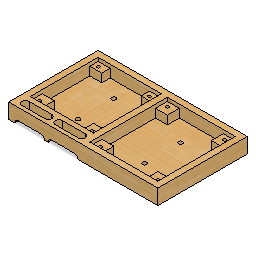
Electronics V8 case (Autodesk Fusion 360 design; units mm, degrees)
Autodesk Fusion 360 part; units mm, degrees
note: some values were not read from the file. Chosen so that the rebuilt part matches the saved one: which face or edge a step refers to.
box "BoxPrimitive1" add length 74.75 width 124.7 height 12.7 placed x (0, 0, -1) y (-1, 0, 0) z (0, 1, 0) at (0, 0, 0) makes body 1
copy_body "CutPasteBodies1" bodies 1 removing the originals makes body 2 in component "Stock"
box "BoxPrimitive1'" add length 52.9 width 56.75 height 8 placed x (0, 0, -1) y (-1, 0, 0) z (0, 1, 0) at (-15.6378, 0, 82.7892) separate body makes body 3 in component "Smaller cutout"
move_body "Move1" bodies 3 to x (1, 0, 0) y (0, 1, 0) z (0, 0, 1) at (-52.3122, 4.7, -82.7892) in component "Smaller cutout"
move_body "Move2" bodies 3 to x (1, 0, 0) y (0, 1, 0) z (0, 0, 1) at (-50, 0, 0) in component "Smaller cutout"
move_body "Move3" bodies 3 to x (1, 0, 0) y (0, 1, 0) z (0, 0, 1) at (50, 0, -21.85) in component "Smaller cutout"
move_body "Move4" bodies 3 to x (1, 0, 0) y (0, 1, 0) z (0, 0, 1) at (5, 0, 5) in component "Smaller cutout"
box "BoxPrimitive1''" add length 64.75 width 56.8 height 5 placed x (0, 0, -1) y (-1, 0, 0) z (0, 1, 0) at (-52.8442, 0, 39.9894) separate body makes body 4 in component "Bigger cutout"
move_body "Move1'" bodies 4 to x (1, 0, 0) y (0, 1, 0) z (0, 0, 1) at (46.6942, 7.7, -44.9894) in component "Bigger cutout"
move_body "Move2'" bodies 4 to x (1, 0, 0) y (0, 1, 0) z (0, 0, 1) at (5, 0, 0) in component "Bigger cutout"
move_body "Move5" bodies 3 to x (0, 0, -1) y (0, 1, 0) z (1, 0, 0) at (-49.95, 0, -189.45) in component "Smaller cutout"
move_body "Move6" bodies 3 to x (1, 0, 0) y (0, 1, 0) z (0, 0, 1) at (-5, 0, 51.75) in component "Smaller cutout"
move_body "Move7" bodies 3 to x (1, 0, 0) y (0, 1, 0) z (0, 0, 1) at (5, 0, 5) in component "Smaller cutout"
move_body "Move3'" bodies 4 to x (1, 0, 0) y (0, 1, 0) z (0, 0, 1) at (-8.85, 0, 0) in component "Bigger cutout"
move_body "Move4'" bodies 4 to x (1, 0, 0) y (0, 1, 0) z (0, 0, 1) at (5, 0, 0) in component "Bigger cutout"
move_face "OffsetFaces1" offset 5 1 faces at (-42.8667, 7.7, -26.5833) on bodies 4 in component "Bigger cutout"
cylinder "CylinderPrimitive1" add diameter 2.5 height 12.7 placed x (1, 0, 0) y (0, 0, -1) z (0, 1, 0) at (-30.8242, 0, 13.5156) separate body makes body 5 in component "PCB screw holes"
copy_body "CopyPasteBodies1" bodies 5 makes body 6 in component "PCB screw holes"
move_body "Move1''" bodies 6 to x (1, 0, 0) y (0, 1, 0) z (0, 0, 1) at (15, 0, 0) in component "PCB screw holes"
copy_body "CopyPasteBodies2" bodies 5 makes body 7 in component "PCB screw holes"
move_body "Move2''" bodies 7 to x (1, 0, 0) y (0, 1, 0) z (0, 0, 1) at (-25, 0, 0) in component "PCB screw holes"
copy_body "CopyPasteBodies3" bodies 5 makes body 8 in component "PCB screw holes"
move_body "Move3''" bodies 8 to x (1, 0, 0) y (0, 1, 0) z (0, 0, 1) at (-50, 0, 0) in component "PCB screw holes"
copy_body "CopyPasteBodies4" bodies 5 makes body 9 in component "PCB screw holes"
move_body "Move4''" bodies 9 to x (1, 0, 0) y (0, 1, 0) z (0, 0, 1) at (-65, 0, 0) in component "PCB screw holes"
copy_body "CopyPasteBodies5" bodies 5 makes body 10 in component "PCB screw holes"
move_body "Move5'" bodies 10 to x (1, 0, 0) y (0, 1, 0) z (0, 0, 1) at (-85, 0, 0) in component "PCB screw holes"
copy_body "CopyPasteBodies6" bodies 5 makes body 11 in component "PCB screw holes"
move_body "Move6'" bodies 11 to x (1, 0, 0) y (0, 1, 0) z (0, 0, 1) at (-105, 0, 0) in component "PCB screw holes"
copy_body "CopyPasteBodies7" bodies 5 makes body 12 in component "PCB screw holes"
move_body "Move7'" bodies 12 to x (1, 0, 0) y (0, 1, 0) z (0, 0, 1) at (30, 0, 0) in component "PCB screw holes"
move_body "Move8" bodies 5 to x (1, 0, 0) y (0, 1, 0) z (0, 0, 1) at (-88.8758, 0, -83.2656) in component "PCB screw holes"
move_body "Move9" bodies 5 to x (1, 0, 0) y (0, 1, 0) z (0, 0, 1) at (3.9, 0, 0) in component "PCB screw holes"
move_body "Move10" bodies 5 to x (1, 0, 0) y (0, 1, 0) z (0, 0, 1) at (0, 0, 3.9) in component "PCB screw holes"
move_body "Move11" bodies 6 to x (1, 0, 0) y (0, 1, 0) z (0, 0, 1) at (-103.8758, 0, -26.5156) in component "PCB screw holes"
move_body "Move12" bodies 6 to x (1, 0, 0) y (0, 1, 0) z (0, 0, 1) at (3.9, 0, 0) in component "PCB screw holes"
move_body "Move13" bodies 6 to x (1, 0, 0) y (0, 1, 0) z (0, 0, 1) at (0, 0, -3.9) in component "PCB screw holes"
move_body "Move14" bodies 7 to x (1, 0, 0) y (0, 1, 0) z (0, 0, 1) at (-10.9758, 0, -83.2656) in component "PCB screw holes"
move_body "Move15" bodies 7 to x (1, 0, 0) y (0, 1, 0) z (0, 0, 1) at (-5.1, 0, 3.9) in component "PCB screw holes"
move_body "Move16" bodies 8 to x (1, 0, 0) y (0, 1, 0) z (0, 0, 1) at (14.0242, 0, -26.5156) in component "PCB screw holes"
move_body "Move17" bodies 8 to x (1, 0, 0) y (0, 1, 0) z (0, 0, 1) at (-5.1, 0, -3.9) in component "PCB screw holes"
move_body "Move18" bodies 9 to x (1, 0, 0) y (0, 1, 0) z (0, 0, 1) at (34.0242, 0, -83.2656) in component "PCB screw holes"
move_body "Move19" bodies 9 to x (1, 0, 0) y (0, 1, 0) z (0, 0, 1) at (3.9, 0, 3.9) in component "PCB screw holes"
move_body "Move20" bodies 10 to x (1, 0, 0) y (0, 1, 0) z (0, 0, 1) at (54.0242, 0, -18.5156) in component "PCB screw holes"
move_body "Move21" bodies 10 to x (1, 0, 0) y (0, 1, 0) z (0, 0, 1) at (3.9, 0, -3.9) in component "PCB screw holes"
move_body "Move22" bodies 11 to x (1, 0, 0) y (0, 1, 0) z (0, 0, 1) at (130.8242, 0, -83.2656) in component "PCB screw holes"
move_body "Move23" bodies 11 to x (1, 0, 0) y (0, 1, 0) z (0, 0, 1) at (-3.9, 0, 3.9) in component "PCB screw holes"
move_body "Move24" bodies 12 to x (1, 0, 0) y (0, 1, 0) z (0, 0, 1) at (-4.1758, 0, -18.5156) in component "PCB screw holes"
move_body "Move25" bodies 12 to x (1, 0, 0) y (0, 1, 0) z (0, 0, 1) at (-3.9, 0, -3.9) in component "PCB screw holes"
move_face "OffsetFaces1'" offset 2 1 faces at (-102.0667, 4.7, -31.9167) on bodies 3 in component "Smaller cutout"
box "BoxPrimitive2" add length 10 width 10 height 7 placed x (0, 0, -1) y (-1, 0, 0) z (0, 1, 0) at (-122.8706, 0, 22.3895) separate body makes body 13 in component "PCB supports"
copy_body "CopyPasteBodies9" bodies 13 makes body 14 in component "PCB supports"
move_body "Move12'" bodies 14 to x (1, 0, 0) y (0, 1, 0) z (0, 0, 1) at (20, 0, 0) in component "PCB supports"
copy_body "CopyPasteBodies10" bodies 13 makes body 15 in component "PCB supports"
move_body "Move13'" bodies 15 to x (1, 0, 0) y (0, 1, 0) z (0, 0, 1) at (35, 0, 0) in component "PCB supports"
copy_body "CopyPasteBodies11" bodies 13 makes body 16 in component "PCB supports"
move_body "Move14'" bodies 16 to x (1, 0, 0) y (0, 1, 0) z (0, 0, 1) at (50, 0, 0) in component "PCB supports"
copy_body "CopyPasteBodies12" bodies 13 makes body 17 in component "PCB supports"
move_body "Move15'" bodies 17 to x (1, 0, 0) y (0, 1, 0) z (0, 0, 1) at (0, 0, -20) in component "PCB supports"
copy_body "CopyPasteBodies13" bodies 13 makes body 18 in component "PCB supports"
move_body "Move16'" bodies 18 to x (1, 0, 0) y (0, 1, 0) z (0, 0, 1) at (0, 0, -40) in component "PCB supports"
copy_body "CopyPasteBodies14" bodies 13 makes body 19 in component "PCB supports"
move_body "Move17'" bodies 19 to x (1, 0, 0) y (0, 1, 0) z (0, 0, 1) at (0, 0, -60) in component "PCB supports"
copy_body "CopyPasteBodies15" bodies 13 makes body 20 in component "PCB supports"
move_body "Move18'" bodies 20 to x (1, 0, 0) y (0, 1, 0) z (0, 0, 1) at (0, 0, -80) in component "PCB supports"
move_body "Move19'" bodies 20 to x (1, 0, 0) y (0, 1, 0) z (0, 0, 1) at (-20, 0, 0) in component "PCB supports"
move_body "Move20'" bodies 20 to x (1, 0, 0) y (0, 1, 0) z (0, 0, 1) at (33.1706, 2.7, -2.1395) in component "PCB supports"
move_body "Move21'" bodies 19 to x (1, 0, 0) y (0, 1, 0) z (0, 0, 1) at (13.1706, 2.7, 24.6105) in component "PCB supports"
move_body "Move22'" bodies 18 to x (1, 0, 0) y (0, 1, 0) z (0, 0, 1) at (56.0706, 2.7, 4.6105) in component "PCB supports"
move_body "Move23'" bodies 17 to x (1, 0, 0) y (0, 1, 0) z (0, 0, 1) at (56.0706, 2.7, -62.1395) in component "PCB supports"
move_body "Move24'" bodies 13 to x (1, 0, 0) y (0, 1, 0) z (0, 0, 1) at (71.0706, 2.7, -27.3895) in component "PCB supports"
move_body "Move25'" bodies 14 to x (1, 0, 0) y (0, 1, 0) z (0, 0, 1) at (51.0706, 2.7, -82.1395) in component "PCB supports"
move_body "Move26" bodies 16 to x (1, 0, 0) y (0, 1, 0) z (0, 0, 1) at (67.8706, 2.7, -27.3895) in component "PCB supports"
move_body "Move27" bodies 15 to x (1, 0, 0) y (0, 1, 0) z (0, 0, 1) at (82.8706, 2.7, -82.1395) in component "PCB supports"
cylinder "CylinderPrimitive1'" add diameter 3.5 height 12.7 placed x (1, 0, 0) y (0, 0, -1) z (0, 1, 0) at (-133.1666, 0, 19.1223) separate body makes body 21 in component "Mounting screw holes"
copy_body "CopyPasteBodies1'" bodies 21 makes body 22 in component "Mounting screw holes"
move_body "Move1'''" bodies 22 to x (1, 0, 0) y (0, 1, 0) z (0, 0, 1) at (25, 0, 0) in component "Mounting screw holes"
copy_body "CopyPasteBodies2'" bodies 21 makes body 23 in component "Mounting screw holes"
move_body "Move2'''" bodies 23 to x (1, 0, 0) y (0, 1, 0) z (0, 0, 1) at (45, 0, 0) in component "Mounting screw holes"
copy_body "CopyPasteBodies3'" bodies 21 makes body 24 in component "Mounting screw holes"
move_body "Move3'''" bodies 24 to x (1, 0, 0) y (0, 1, 0) z (0, 0, 1) at (75, 0, 0) in component "Mounting screw holes"
move_body "Move4'''" bodies 21 to x (1, 0, 0) y (0, 1, 0) z (0, 0, 1) at (39.9166, 0, -60.4973) in component "Mounting screw holes"
move_body "Move5''" bodies 21 to x (1, 0, 0) y (0, 1, 0) z (0, 0, 1) at (0, 0, -15) in component "Mounting screw holes"
move_body "Move6''" bodies 22 to x (1, 0, 0) y (0, 1, 0) z (0, 0, 1) at (14.9166, 0, -60.4973) in component "Mounting screw holes"
move_body "Move7''" bodies 22 to x (1, 0, 0) y (0, 1, 0) z (0, 0, 1) at (0, 0, 15) in component "Mounting screw holes"
move_body "Move8'" bodies 23 to x (1, 0, 0) y (0, 1, 0) z (0, 0, 1) at (54.7666, 0, -56.4973) in component "Mounting screw holes"
move_body "Move9'" bodies 23 to x (1, 0, 0) y (0, 1, 0) z (0, 0, 1) at (0, 0, -15) in component "Mounting screw holes"
move_body "Move10'" bodies 24 to x (1, 0, 0) y (0, 1, 0) z (0, 0, 1) at (24.7666, 0, -56.4973) in component "Mounting screw holes"
move_body "Move11'" bodies 24 to x (1, 0, 0) y (0, 1, 0) z (0, 0, 1) at (0, 0, 15) in component "Mounting screw holes"
combine "Combine1" operation cut target body 2 tool bodies 3 4 keep tools result as body 25 in component "Dished out"
combine "Combine1'" operation add target body 25 tool bodies 13 14 15 16 17 18 19 20 keep tools result as body 26 in component "Dished out, with supports"
combine "Combine1''" operation cut target body 26 tool bodies 5 6 7 8 9 10 11 12 21 22 23 24 keep tools result as body 27 in component "Tray with screw holes"
box "BoxPrimitive1'''" add length 6 width 25 height 12.7 placed x (0, 0, 1) y (1, 0, 0) z (0, 1, 0) at (-104.7132, 0, 18.6921) separate body makes body 28 in component "Cable support cutout"
fillet "Fillet1" radius 3 4 edges at (-104.7132, 6.35, 24.6921) (-104.7132, 6.35, 18.6921) (-79.7132, 6.35, 24.6921) (-79.7132, 6.35, 18.6921) on bodies 28 in component "Cable support cutout"
copy_body "CopyPasteBodies1''" bodies 28 makes body 29 in component "Cable support cutout"
move_body "Move1''''" bodies 29 to x (1, 0, 0) y (0, 1, 0) z (0, 0, 1) at (45, 0, 0) in component "Cable support cutout"
move_body "Move2''''" bodies 28 to x (1, 0, 0) y (0, 1, 0) z (0, 0, 1) at (-19.9868, 0, -21.6921) in component "Cable support cutout"
move_body "Move3''''" bodies 28 to x (1, 0, 0) y (0, 1, 0) z (0, 0, 1) at (5, 0, -6) in component "Cable support cutout"
move_body "Move4''''" bodies 29 to x (1, 0, 0) y (0, 1, 0) z (0, 0, 1) at (-37.9868, 0, -27.6921) in component "Cable support cutout"
move_body "Move5'''" bodies 29 to x (1, 0, 0) y (0, 1, 0) z (0, 0, 1) at (6, 0, 0) in component "Cable support cutout"
combine "Combine1'''" operation cut target body 27 tool bodies 28 29 keep tools result as body 30 in component "Nearly completed unit"
copy_body "CopyPasteBodies1'''" bodies 28 makes body 31 in component "holder cutout"
move_body "Move1'''''" bodies 31 to x (1, 0, 0) y (0, 0, 1) z (0, -1, 0) at (0, -9, -9) in component "holder cutout"
copy_body "CopyPasteBodies2''" bodies 29 makes body 32 in component "holder cutout"
move_body "Move2'''''" bodies 32 to x (1, 0, 0) y (0, 0, 1) z (0, -1, 0) at (0, -9, -9) in component "holder cutout"
move_body "Move3'''''" bodies 31 32 to x (1, 0, 0) y (0, 1, 0) z (0, 0, 1) at (0, 3, 0) in component "holder cutout"
move_body "Move4'''''" bodies 31 32 to x (1, 0, 0) y (0, 1, 0) z (0, 0, 1) at (0, 0, -3) in component "holder cutout"
move_body "Move5''''" bodies 31 32 to x (1, 0, 0) y (0, 1, 0) z (0, 0, 1) at (0, 0, 5) in component "holder cutout"
combine "Combine1''''" operation cut target body 30 tool bodies 31 32 keep tools result as body 33 in component "Completed unit"
move_face "OffsetFaces1''" offset -3 1 faces at (-113.0333, 5.0333, -59.75) on bodies 33 in component "Completed unit"
move_face "OffsetFaces2" offset -3 1 faces at (-73.4667, 5.0333, -59.75) on bodies 33 in component "Completed unit"
move_face "MoveFace1" to x (1, 0, 0) y (0, 1, 0) z (0, 0, 1) at (-0.9998, 0, 1.0002) 1 faces at (-71.5019, 6.4667, -67.0349) on bodies 33 in component "Completed unit"
move_face "MoveFace2" to x (1, 0, 0) y (0, 1, 0) z (0, 0, 1) at (0, 0, -1) 1 faces at (-116.1981, 3.2333, -15.7151) on bodies 33 in component "Completed unit"
move_face "MoveFace3" to x (1, 0, 0) y (0, 1, 0) z (0, 0, 1) at (-1, 0, 0) 1 faces at (-72.2981, 3.2333, -15.7151) on bodies 33 in component "Completed unit"
move_face "MoveFace4" to x (1, 0, 0) y (0, 1, 0) z (0, 0, 1) at (-1, 0, 1) 1 faces at (-10.1113, 3.2333, -65.5416) on bodies 33 in component "Completed unit"
move_face "MoveFace5" to x (1, 0, 0) y (0, 1, 0) z (0, 0, 1) at (1, 0, -1) 1 faces at (-56.6562, 3.2333, -8.7755) on bodies 33 in component "Completed unit"
move_face "MoveFace6" to x (1, 0, 0) y (0, 1, 0) z (0, 0, 1) at (1, 0, 1) 1 faces at (-56.6887, 3.2333, -66.1584) on bodies 33 in component "Completed unit"
move_face "MoveFace7" to x (1, 0, 0) y (0, 1, 0) z (0, 0, 1) at (0, 0, 1) 1 faces at (-115.4019, 6.4667, -19.0849) on bodies 33 in component "Completed unit"
move_face "MoveFace8" to x (1, 0, 0) y (0, 1, 0) z (0, 0, 1) at (1, 0, 0) 1 faces at (-73.2981, 3.2333, -15.7151) on bodies 33 in component "Completed unit"
move_face "MoveFace9" to x (1, 0, 0) y (0, 1, 0) z (0, 0, 1) at (-0.0002, 0, -1.0002) 1 faces at (-72.5017, 6.4667, -66.0348) on bodies 33 in component "Completed unit"
move_face "MoveFace10" to x (1, 0, 0) y (0, 1, 0) z (0, 0, 1) at (0, 0, 1) 1 faces at (-55.6562, 6.4667, -9.7755) on bodies 33 in component "Completed unit"
move_face "MoveFace11" to x (1, 0, 0) y (0, 1, 0) z (0, 0, 1) at (0, 0, -1) 1 faces at (-8.6887, 3.2333, -65.1584) on bodies 33 in component "Completed unit"
move_face "MoveFace12" to x (1, 0, 0) y (0, 1, 0) z (0, 0, 1) at (-1, 0, -1) 1 faces at (-55.6887, 3.2333, -65.1584) on bodies 33 in component "Completed unit"
component "Archive" placed x (1, 0, 0) y (0, 1, 0) z (0, 0, 1) at (0, 0, 0)
component "Completed unit" placed x (1, 0, 0) y (0, 1, 0) z (0, 0, 1) at (0, 0, 0)
component "Stock" placed x (1, 0, 0) y (0, 1, 0) z (0, 0, 1) at (0, 0, 0) in component "Archive"
component "Smaller cutout" placed x (1, 0, 0) y (0, 1, 0) z (0, 0, 1) at (0, 0, 0) in component "Archive"
component "Bigger cutout" placed x (1, 0, 0) y (0, 1, 0) z (0, 0, 1) at (0, 0, 0) in component "Archive"
component "Dished out" placed x (1, 0, 0) y (0, 1, 0) z (0, 0, 1) at (0, 0, 0) in component "Archive"
component "PCB supports" placed x (1, 0, 0) y (0, 1, 0) z (0, 0, 1) at (0, 0, 0) in component "Archive"
component "Dished out, with supports" placed x (1, 0, 0) y (0, 1, 0) z (0, 0, 1) at (0, 0, 0) in component "Archive"
component "Mounting screw holes" placed x (1, 0, 0) y (0, 1, 0) z (0, 0, 1) at (0, 0, 0) in component "Archive"
component "PCB screw holes" placed x (1, 0, 0) y (0, 1, 0) z (0, 0, 1) at (0, 0, 0) in component "Archive"
component "Cable support cutout" placed x (1, 0, 0) y (0, 1, 0) z (0, 0, 1) at (0, 0, 0) in component "Archive"
component "Tray with screw holes" placed x (1, 0, 0) y (0, 1, 0) z (0, 0, 1) at (0, 0, 0) in component "Archive"
component "holder cutout" placed x (1, 0, 0) y (0, 1, 0) z (0, 0, 1) at (0, 0, 0) in component "Archive"
component "Nearly completed unit" placed x (1, 0, 0) y (0, 1, 0) z (0, 0, 1) at (0, 0, 0) in component "Archive"
